Autodesk Inventor part; units mm, degrees
(part 2 of 2)
  spline S221 degree 2 poles (-29.3161, 1.0228) (-29.3161, 1.3194) (-29.0838, 1.8433) (-28.8564, 2.0361) knots 0 0 0 1 2 2 2
  spline S222 degree 2 poles (-28.8564, 2.0361) (-28.6141, 2.2388) (-27.9962, 2.4514) (-27.5266, 2.4514) knots 0 0 0 1 2 2 2
  spline S223 degree 2 poles (-31.2687, 2.4514) (-30.809, 2.4514) (-30.0131, 2.2042) (-29.7511, 2.0658) knots 0 0 0 1 2 2 2
  line L360 (-29.7511, 2.0658) -> (-29.7511, 1.2007)
  line L361 (-29.7511, 1.2007) -> (-29.7906, 1.2007)
  spline S224 degree 2 poles (-29.7906, 1.2007) (-29.8895, 1.2798) (-30.1564, 1.4677) (-30.3789, 1.5715) knots 0 0 0 1 2 2 2
  spline S225 degree 2 poles (-30.3789, 1.5715) (-30.5717, 1.6654) (-31.0462, 1.8038) (-31.2983, 1.8038) knots 0 0 0 1 2 2 2
  spline S226 degree 2 poles (-31.2983, 1.8038) (-31.4812, 1.8038) (-31.9014, 1.7198) (-32.0003, 1.6506) knots 0 0 0 1 2 2 2
  spline S227 degree 2 poles (-32.0003, 1.6506) (-32.1436, 1.5566) (-32.2722, 1.3441) (-32.2722, 1.1266) knots 0 0 0 1 2 2 2
  spline S228 degree 2 poles (-32.2722, 1.1266) (-32.2722, 0.8547) (-31.9756, 0.5729) (-31.5949, 0.479) knots 0 0 0 1 2 2 2
  spline S229 degree 2 poles (-31.5949, 0.479) (-31.4466, 0.4444) (-30.9721, 0.3455) (-30.7694, 0.2912) knots 0 0 0 1 2 2 2
  spline S230 degree 2 poles (-30.7694, 0.2912) (-30.2454, 0.1379) (-29.7709, -0.4948) (-29.7709, -0.9447) knots 0 0 0 1 2 2 2
  spline S231 degree 2 poles (-29.7709, -0.9447) (-29.7709, -1.5675) (-30.7051, -2.3436) (-31.4763, -2.3436) knots 0 0 0 1 2 2 2
  spline S232 degree 2 poles (-31.4763, -2.3436) (-31.8569, -2.3436) (-32.6281, -2.1558) (-32.8901, -2.0124) knots 0 0 0 1 2 2 2
  line L362 (-32.8901, -2.0124) -> (-32.8901, -1.1869)
  line L363 (-32.8901, -1.1869) -> (-32.8505, -1.1869)
  spline S233 degree 2 poles (-32.8505, -1.1869) (-32.5539, -1.4242) (-31.8322, -1.696) (-31.4615, -1.696) knots 0 0 0 1 2 2 2
  spline S234 degree 2 poles (-31.4615, -1.696) (-31.0808, -1.696) (-30.5568, -1.3747) (-30.5568, -1.0534) knots 0 0 0 1 2 2 2
  spline S235 degree 2 poles (-30.5568, -1.0534) (-30.5568, -0.7618) (-30.8683, -0.48) (-31.2143, -0.391) knots 0 0 0 1 2 2 2
  spline S236 degree 2 poles (-31.2143, -0.391) (-31.3824, -0.3465) (-31.8075, -0.2575) (-32.0398, -0.2032) knots 0 0 0 1 2 2 2
  spline S237 degree 2 poles (-32.0398, -0.2032) (-32.544, -0.0746) (-33.0581, 0.5136) (-33.0581, 1.0228) knots 0 0 0 1 2 2 2
  spline S238 degree 2 poles (-33.0581, 1.0228) (-33.0581, 1.3194) (-32.8258, 1.8433) (-32.5984, 2.0361) knots 0 0 0 1 2 2 2
  spline S239 degree 2 poles (-32.5984, 2.0361) (-32.3562, 2.2388) (-31.7383, 2.4514) (-31.2687, 2.4514) knots 0 0 0 1 2 2 2
  point P0 (0, 0)
  dimension "d26" = 80
  dimension "d27" = 40
  dimension "d29" = 10
  dimension "d30" = 5
  dimension "d33" = 80
  dimension "d34" = 15
  dimension "d35" = 2.5
  dimension "d36" = 40
  constraints: 4 other
  measures "d26" distance between parallel lines of L3 L1
  measures "d27" distance from line of point (0, 0) L1
  measures "d29" distance of L0.end L1.end
  measures "d30" distance between parallel lines of L4 L0
  measures "d33" distance of L6.end L7.end
  measures "d34" distance of L5.end L6.end
  measures "d35" distance between parallel lines of L9 L7
  measures "d36" distance from line of point (0, 0) L6
emboss "Emboss1" sketch "Sketch3" operation cut depth 1 direction (0, 1, 0) wrap yes faces at (74.675, 58.7251, -13.3333)
equation "\"d2\" = Diameter_1"
equation "\"d6\" = 0.25 * d2 + 0.25 * d3"
equation "\"d27\" = 0.5 * d26"
equation "\"d36\" = 0.5 * d33"
equation "\"Diameter_1\" = 190"
body "Solid1"
